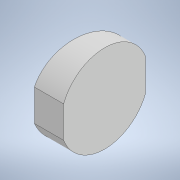
# Autodesk Inventor part: 711123
Saved by Autodesk Inventor 2022 (Build 260153000, 153)
## iProperties
Created: 2021-10-21
Part Number: 711123
Material: Типовые
Document SubType Name: Modeling
Designer: RaNSiD
Density: 1 g/cm^3
Appearance: По умолчанию
Author: RaNSiD
Autodesk Inventor part; units mm, degrees
ref_plane "YZ Plane" through (0, 0, 0) normal (1, 0, 0) x (0, 1, 0)
ref_plane "XY Plane" through (0, 0, 0) normal (0, 0, 1) x (1, 0, 0)
sketch "Эскиз1" plane through (0, 0, 0) normal (0, 0, 1) x (1, 0, 0)
  line L0 (0, 0) -> (20, 0)
  line L1 (20, 0) -> (20, 30)
  line L2 (20, 30) -> (0, 30)
  line L3 (0, 30) -> (0, 0)
  dimension "d0" = 20
  dimension "d1" = 30
  constraints: 8 end point, 2 parallel, 1 horizontal, 1 perpendicular
  measures "d0" distance of L2.end L1.end
  measures "d1" distance of L1.end L0.end
revolve "Вращение1" add sketch "Эскиз1" angle 360 about axis through (0, 0, 0) along (1, 0, 0)
sketch "Эскиз2" plane through (0, 0, 0) normal (-1, 0, 0) x (0, 0, 1)
  circle A0 centre (0, 0) radius 26
  dimension "d3" = 52
  constraints: 1 centre point, 1 coincident
  measures "d3" diameter of A0
extrude "Выдавливание1" cut sketch "Эскиз2" against normal blind 16
sketch "Эскиз3" plane through (0, 0, 0) normal (-1, 0, 0) x (0, 0, 1)
  line L0 (28, -30) -> (-28, -30)
  line L1 (-28, -30) -> (-28, 30)
  line L2 (-28, 30) -> (28, 30)
  line L3 (28, 30) -> (28, -30)
  circle A0 centre (0, 0) radius 30 construction
  point P0 (0, 30)
  dimension "d6" = 56
  constraints: 8 end point, 2 parallel, 2 tangent, 1 horizontal, 1 midpoint, 1 perpendicular, 1 vertical alignment
  measures "d6" distance of L1.end L2.end
extrude "Выдавливание2" cut sketch "Эскиз3" against normal blind 20 keep common part
ref_plane "РабПлоскость1" through (0, 30, 0) normal (0, 1, 0) x (-1, 0, 0)
sketch "Эскиз4" plane through (0, 30, 0) normal (0, 1, 0) x (-1, 0, 0)
  line L0 (-20, 28) -> (0, 28) construction
  line L1 (0, -28) -> (-20, -28) construction
  line L2 (0, -28) -> (0, 28) construction
  line L3 (-20, 28) -> (0, 28) projected
  line L4 (-20, -28) -> (-20, 28) construction
  line L5 (0, 28) -> (0, -28) projected
  line L6 (0, 28) -> (-9.8743, -28)
  line L7 (0, -28) -> (-20, -28) projected
  line L8 (0, -28) -> (-9.8743, -28)
  line L9 (0, -28) -> (0, 28)
  point P0 (0, 0)
  dimension "d10" = 10
  constraints: 6 end point, 1 collinear, 1 point on line
  measures "d10" angle of L6 L2
extrude "Выдавливание3" cut sketch "Эскиз4" against normal blind 60
